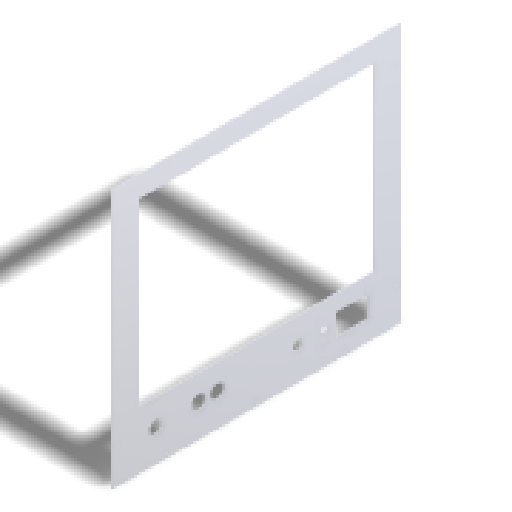
# Autodesk Inventor part: Front Panel
Saved by Autodesk Inventor 2023.2 (Build 272271000, 271)
## iProperties
Created: 2023-02-06
Part Number: Front Panel
Material: Aluminum 6061
Document SubType Name: Modeling
Designer: remop
Density: 2.7 g/cm^3
Appearance: Aluminum - Flat
Author: remop
Autodesk Inventor part; units mm, degrees
ref_plane "YZ Plane" through (0, 0, 0) normal (1, 0, 0) x (0, 1, 0)
ref_plane "XZ Plane" through (0, 0, 0) normal (0, 1, 0) x (-1, 0, 0)
ref_plane "XY Plane" through (0, 0, 0) normal (0, 0, 1) x (1, 0, 0)
sketch "Sketch1" plane through (0, 0, 0) normal (1, 0, 0) x (0, 1, 0)
  line L0 (465, 411) -> (465, -123) projected
  line L1 (465, -123) -> (-15, -123) projected
  line L2 (-15, -123) -> (-15, 411) projected
  line L3 (-15, 411) -> (465, 411) projected
  circle A0 centre (400, -113.5) radius 1.75 projected
  circle A1 centre (50, 401.5) radius 1.75 projected
  circle A2 centre (400, 401.5) radius 1.75 projected
  circle A3 centre (-7.5, -21) radius 1.75 projected
  circle A4 centre (-7.5, 144) radius 1.75 projected
  circle A5 centre (-7.5, 309) radius 1.75 projected
  circle A6 centre (457.5, 144) radius 1.75 projected
  circle A7 centre (457.5, -21) radius 1.75 projected
  circle A8 centre (457.5, 309) radius 1.75 projected
  circle A9 centre (50, -113.5) radius 1.75 projected
  circle A10 centre (408.5, -78.0001) radius 1.75 projected
  circle A11 centre (415.5, -88.0001) radius 1.75 projected
  circle A12 centre (408.5, -88.0001) radius 1.75 projected
  circle A13 centre (415.5, -78.0001) radius 1.75 projected
  line L4 (47, 380) -> (15, 380) projected
  line L5 (15, 380) -> (15, 352) projected
  line L6 (15, 352) -> (47, 352) projected
  line L7 (47, 352) -> (47, 380) projected
  circle A14 centre (31, 384) radius 1.6 projected
  circle A15 centre (31, 348) radius 1.6 projected
  line L8 (40.5, 334.5) -> (21.5, 334.5) projected
  line L9 (21.5, 334.5) -> (21.5, 321.5) projected
  line L10 (21.5, 321.5) -> (40.5, 321.5) projected
  line L11 (40.5, 321.5) -> (40.5, 334.5) projected
  circle A16 centre (63, 292) radius 1.75 projected
  circle A17 centre (63, 12) radius 1.75 projected
  circle A18 centre (63, 62) radius 1.75 projected
  circle A19 centre (38, 37) radius 29.5 projected
  circle A20 centre (13, 292) radius 1.75 projected
  circle A21 centre (63, 242) radius 1.75 projected
  circle A22 centre (13, 12) radius 1.75 projected
  circle A23 centre (13, 62) radius 1.75 projected
  circle A24 centre (13, 242) radius 1.75 projected
  circle A25 centre (38, 267) radius 29.5 projected
  circle A26 centre (25, -23) radius 12.5 projected
  circle A27 centre (37, -73.5) radius 1.25 projected
  circle A28 centre (13, -92.5) radius 1.25 projected
  circle A29 centre (13, -32.5) radius 1.25 projected
  circle A30 centre (25, -53) radius 12.5 projected
  circle A31 centre (13, -62.5) radius 1.25 projected
  circle A32 centre (37, -13.5) radius 1.25 projected
  circle A33 centre (37, -43.5) radius 1.25 projected
  circle A34 centre (25, -83) radius 12.5 projected
  circle A35 centre (265, 270.25) radius 1.6 projected
  circle A36 centre (240, 295.25) radius 1.6 projected
  circle A37 centre (265, -7.25) radius 1.6 projected
  circle A38 centre (240, -7.25) radius 1.6 projected
  circle A39 centre (240, 17.75) radius 1.6 projected
  circle A40 centre (265, 17.75) radius 1.6 projected
  circle A41 centre (265, 295.25) radius 1.6 projected
  circle A42 centre (240, 270.25) radius 1.6 projected
  point P0 (0, 0)
  point P1 (37, 276.8868)
  point P2 (37, 271.1132)
  constraints: 1 other
extrude "Extrusion1" add sketch "Sketch1" along normal blind 2 contours L0 L1 L2 L3 | A10 | A11 | A12 | A13 | L7 L6 L5 L4 | A14 | A15 | L11 L10 L9 L8 | A16 | A17 | A18 | A19 | A20 | A21 | A22 | A23 | A24 | A25 | A26 | A27 | A28 | A29 | A30 | A31 | A32 | A33 | A34 | A35 | A36 | A37 | A38 | A39 | A40 | A41 | A42
sketch "Sketch2" plane through (0, 0, 0) normal (-1, 0, 0) x (0, 0, 1)
  line L0 (411, -15) -> (-123, -15) projected
  line L1 (411, 465) -> (411, -15) projected
  line L2 (-123, 465) -> (411, 465) projected
  line L3 (-123, -15) -> (-123, 465) projected
  circle A0 centre (-113.5, 50) radius 1.75 projected
  circle A1 centre (-21, 457.5) radius 1.75 projected
  circle A2 centre (144, 457.5) radius 1.75 projected
  circle A3 centre (309, -7.5) radius 1.75 projected
  circle A4 centre (144, -7.5) radius 1.75 projected
  circle A5 centre (-21, -7.5) radius 1.75 projected
  circle A6 centre (401.5, 400) radius 1.75 projected
  circle A7 centre (401.5, 50) radius 1.75 projected
  circle A8 centre (-113.5, 400) radius 1.75 projected
  circle A9 centre (309, 457.5) radius 1.75 projected
  line L4 (-73, 425) -> (361, 425)
  line L5 (361, 425) -> (361, 92)
  line L6 (361, 92) -> (-73, 92)
  line L7 (-73, 92) -> (-73, 425)
  point P0 (0, 0)
  dimension "d2" = 50
  dimension "d3" = 50
  dimension "d4" = 40
  dimension "d5" = 107
  constraints: 8 end point, 2 parallel, 1 horizontal, 1 perpendicular
  measures "d2" distance between parallel lines of L3 L7
  measures "d3" distance between parallel lines of L1 L5
  measures "d4" distance between parallel lines of L2 L4
  measures "d5" distance between parallel lines of L0 L6
extrude "Extrusion2" cut sketch "Sketch2" against normal blind 2 contours L4 L5 L6 L7
sketch "Sketch3" plane through (0, 0, 0) normal (-1, 0, 0) x (0, 0, 1)
  line L0 (361, 425) -> (361, 92) projected
  line L1 (361, 92) -> (-73, 92) projected
  line L2 (-73, 92) -> (-73, 425) projected
  line L3 (-73, 425) -> (361, 425) projected
  line L4 (411, -15) -> (-123, -15) projected
  line L5 (411, 465) -> (411, -15) projected
  line L6 (-123, 465) -> (411, 465) projected
  line L7 (-123, -15) -> (-123, 465) projected
  circle A0 centre (-113.5, 50) radius 1.75 projected
  circle A1 centre (-21, 457.5) radius 1.75 projected
  circle A2 centre (144, 457.5) radius 1.75 projected
  circle A3 centre (309, -7.5) radius 1.75 projected
  circle A4 centre (144, -7.5) radius 1.75 projected
  circle A5 centre (-21, -7.5) radius 1.75 projected
  circle A6 centre (401.5, 400) radius 1.75 projected
  circle A7 centre (401.5, 50) radius 1.75 projected
  circle A8 centre (-113.5, 400) radius 1.75 projected
  circle A9 centre (309, 457.5) radius 1.75 projected
  circle A10 centre (331, 45) radius 11.5
  line L8 (-60.221, 60.412) -> (-3.121, 60.412) construction
  line L9 (-60.221, 22.612) -> (-60.221, 60.412) construction
  line L10 (-3.121, 22.612) -> (-60.221, 22.612) construction
  line L11 (-3.121, 39.012) -> (-3.121, 22.612) construction
  line L12 (-3.121, 50.012) -> (-3.121, 39.012) construction
  line L13 (-3.121, 60.412) -> (-3.121, 50.012) construction
  arc A11 (-4.921, 57.812) -> (-5.721, 58.612) centre (-5.721, 57.812) ccw construction
  line L14 (-4.921, 30.612) -> (-4.921, 57.812) construction
  arc A12 (-5.721, 29.812) -> (-4.921, 30.612) centre (-5.721, 30.612) ccw construction
  line L15 (-57.621, 29.812) -> (-5.721, 29.812) construction
  arc A13 (-58.421, 30.612) -> (-57.621, 29.812) centre (-57.621, 30.612) ccw construction
  line L16 (-58.421, 57.812) -> (-58.421, 30.612) construction
  arc A14 (-57.621, 58.612) -> (-58.421, 57.812) centre (-57.621, 57.812) ccw construction
  line L17 (-5.721, 58.612) -> (-57.621, 58.612) construction
  circle A15 centre (18.046, 27) radius 1.75 construction
  circle A16 centre (18.0461, 44.7969) radius 3.5 construction
  circle A17 centre (18.0461, 44.7969) radius 4.5
  circle A18 centre (18.046, 27) radius 2.5
  line L18 (-61.221, 61.412) -> (-2.121, 61.412)
  line L19 (-2.121, 61.412) -> (-2.121, 21.612)
  line L20 (-2.121, 21.612) -> (-61.221, 21.612)
  line L21 (-61.221, 21.612) -> (-61.221, 61.412)
  circle A19 centre (-65, 62) radius 1.6 projected
  circle A20 centre (-65, 21) radius 1.6 projected
  circle A21 centre (28, 62) radius 1.6 projected
  circle A22 centre (28, 21) radius 1.6 projected
  circle A23 centre (251, 45) radius 12.5
  circle A24 centre (241.5, 57) radius 1.25
  circle A25 centre (260.5, 33) radius 1.25
  circle A26 centre (225.5, 33) radius 1.25
  circle A27 centre (206.5, 57) radius 1.25
  circle A28 centre (216, 45) radius 12.5
  circle A29 centre (68.0461, 45) radius 8
  point P0 (0, 0)
  dimension "d11" = 23
  dimension "d12" = 60
  dimension "d13" = 80
  dimension "d16" = 9
  dimension "d17" = 5
  dimension "d18" = 1
  dimension "d19" = 1
  dimension "d20" = 1
  dimension "d21" = 1
  dimension "d22" = 9.5
  dimension "d23" = 9.5
  dimension "d24" = 12
  dimension "d25" = 12
  dimension "d26" = 25
  dimension "d27" = 2.5
  dimension "d30" = 35
  dimension "d35" = 80
  dimension "d36" = 16
  dimension "d37" = 50
  constraints: 10 centre point, 8 end point, 2 coincident, 2 horizontal, 2 horizontal alignment, 2 parallel, 1 equal radius, 1 perpendicular, 6 other
  measures "d11" diameter of A10
  measures "d12" distance from line of L4 A10.centre
  measures "d13" distance from line of L5 A10.centre
  measures "d16" diameter of A17
  measures "d17" diameter of A18
  measures "d18" distance between parallel lines of L8 L18
  measures "d19" distance between parallel lines of L21 L9
  measures "d20" distance between parallel lines of L19 L12
  measures "d21" distance between parallel lines of L10 L20
  measures "d22" horizontal distance of A24.centre A23.centre
  measures "d23" horizontal distance of A25.centre A23.centre
  measures "d24" vertical distance of A24.centre A23.centre
  measures "d25" vertical distance of A23.centre A25.centre
  measures "d26" diameter of A23
  measures "d27" diameter of A25
  measures "d30" distance of A25.centre A26.centre
  measures "d35" distance of A10.centre A23.centre
  measures "d36" diameter of A29
  measures "d37" horizontal distance of A16.centre A29.centre
extrude "Extrusion3" cut sketch "Sketch3" against normal through all contours A10 | A17 | A18 | L18 L19 L20 L21 | A19 | A20 | A21 | A22 | A23 | A24 | A25 | A26 | A27 | A28 | A29
equation "\"d3\" = d2"
equation "\"d19\" = d18"
equation "\"d20\" = d19"
equation "\"d21\" = d19"
equation "\"d23\" = d22"
equation "\"d25\" = d24"
body "Solid1"
